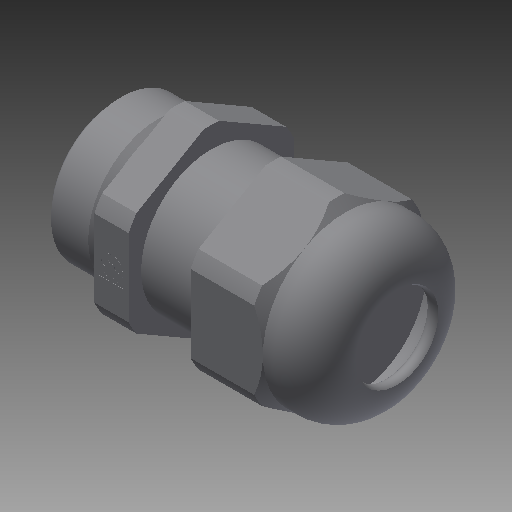
# Autodesk Inventor part: SKINTOP ST PG 13,5      Art. Nr. 53015030(F=5) Kunststoff
Saved by Autodesk Inventor 2019.3 (Build 233278000, 278)
## iProperties
Category: PARTsolutions
Company: LAPP
Created: 2018-12-13
Part Number: SKINTOP ST PG 13,5      Art. Nr. 53015030(F=5) Kunststoff
Material: Generic
Catalog Web Link: www.cadenas.de
Description: SKINTOP® ST-Cable gland plastic
Vendor: LAPP
Document SubType Name: Modeling
Designer: psadmin
Manufacturer: LAPP
Mass: 14.2643 g
Surface Area: 52.1864 cm^2
Volume: 14.2643 cm^3
Density: 1 g/cm^3
Appearance: PSOLRGB-175-175-175
PSOL_IDENT_0: {$CADENAS_DATA\23d-libs\lapp_kabel\skintop_kabelverschraubungen\skintop_kabelverschraubungen_polyami
PSOL_IDENT_1: d_pg\skintop_kabelverschraubungen_polyamid_pg\st_pg.prj},235 {VTYP=3D},{NB=SKINTOP ST PG 13,5      A
PSOL_IDENT_2: rt. Nr. 53015030(F=5)},{LINA=SKINTOP ST PG 13,5      Art. Nr. 53015030},{NN=SKINTOP® ST},{DATE=06.12
PSOL_IDENT_3: .2018 13:21:11},{GEOMDATE=18.12.2013 09:14:44},{VERSION=},{LINEID=100},{WBVAR=F},{WBNUMERIC=F}  {NB=
PSOL_IDENT_4: SKINTOP ST PG 13,5      Art. Nr. 53015030(F=5)},{LINA=SKINTOP ST PG 13,5      Art. Nr. 53015030},{KT=
PSOL_IDENT_5: DUMMY},{IDNR=},{ATN=53015030},{PG=PG 13,5},{ID=0.000},{RS=0.000},{FMIN=5.0},{FMAX=12.0},{F=5},{NDM=2
PSOL_IDENT_6: 0.4},{X=9},{SW=24},{A=26.5},{C=41.0},{D=9.0},{E=18.0},{H=10.5},{J=6.0},{K=5.0},{L=20.4},{XMAX=9},{RA
PSOL_IDENT_7: L7001=X},{RAL7035=},{RAL9005=},{MATERIAL=Kunststoff},{VPE=MIN}
NN: SKINTOP® ST
NT: Cable gland plastic
NB: SKINTOP® ST PG 13,5      Art. Nr. 53015030(F=5)
NBSYN: SKINTOP® ST $PG.      Art. Nr. $ATN.(F=$F.)
LINA: SKINTOP® ST PG 13,5      Art. Nr. 53015030
ATN: 53015030
PG: PG 13,5
FMIN: 5
FMAX: 12
F: 5
SW: 24
A: 26.5
C: 41
D: 9
RAL7001: X
MATERIAL: Plastic
VPE: 0
SUPPLIER: LAPP
ARTICLENO: SKINTOP ST PG 13,5      Art. Nr. 53015030(F=5)
BOMINFO: SKINTOP ST PG 13,5      Art. Nr. 53015030
CREATOR: CADENAS GmbH
Title: SKINTOP ST PG 13,5      Art. Nr. 53015030
Author: Cadenas PARTsolutions
Comments: Cable gland plastic
Autodesk Inventor part; units mm, degrees
ref_plane "YZ Plane" through (0, 0, 0) normal (1, 0, 0) x (0, 1, 0)
ref_plane "XZ Plane" through (0, 0, 0) normal (0, 1, 0) x (-1, 0, 0)
ref_plane "XY Plane" through (0, 0, 0) normal (0, 0, 1) x (1, 0, 0)
sketch "Sketch_1" plane through (0, 0, 0) normal (0, 0, 1) x (1, 0, 0)
  line L0 (41, 0) -> (0, 0)
  line L1 (0, 8.92) -> (0, 3.27)
  arc A0 (0, 3.27) -> (0.77, 2.5) centre (0.77, 3.27) ccw
  line L2 (0.77, 2.5) -> (35, 2.5)
  line L3 (35, 2.5) -> (35, 10.2)
  arc A1 (39.1884, 6.3116) -> (35, 10.2) centre (35, 6) ccw
  arc A2 (39.1884, 6.3116) -> (41, 6) centre (40.225, 6.9162) ccw
  arc A3 (41, 6) -> (35, 12) centre (35, 6) ccw
  line L4 (35, 12) -> (33.5, 12)
  line L5 (33.5, 12) -> (29.5, 16)
  line L6 (29.5, 16) -> (23, 16)
  line L7 (23, 16) -> (23, 10.2)
  line L8 (23, 10.2) -> (14, 10.2)
  line L9 (14, 10.2) -> (14, 16)
  line L10 (14, 16) -> (9, 16)
  line L11 (9, 16) -> (9, 9.69)
  line L12 (9, 9.69) -> (7.2, 9.69)
  line L13 (7.2, 9.69) -> (6.3167, 10.2)
  line L14 (6.3167, 10.2) -> (0.9, 10.2)
  line L15 (0.9, 10.2) -> (0.9, 9.69)
  line L16 (0.9, 9.69) -> (0.77, 9.69)
  arc A4 (0.77, 9.69) -> (0, 8.92) centre (0.77, 8.92) ccw
  constraints: 34 end point, 10 point on circle, 5 centre point
revolve "Revolution1" add sketch "Sketch_1" angle 360 about axis through (41, 0, 0) along (-1, 0, 0)
sketch "Sketch_2" plane through (9, 0, 0) normal (1, 0, 0) x (0, 0, -1)
  line L0 (-24, 24) -> (-24, -24)
  line L1 (-24, -24) -> (24, -24)
  line L2 (24, -24) -> (24, 24)
  line L3 (24, 24) -> (-24, 24)
  arc A0 (-12, -5.6181) -> (-10.8654, -7.5833) centre (0, 0) ccw
  line L4 (-10.8654, -7.5833) -> (-1.1346, -13.2013)
  arc A1 (-1.1346, -13.2013) -> (1.1346, -13.2013) centre (0, 0) ccw
  line L5 (1.1346, -13.2013) -> (10.8654, -7.5833)
  arc A2 (10.8654, -7.5833) -> (12, -5.6181) centre (0, 0) ccw
  line L6 (12, -5.6181) -> (12, 5.6181)
  arc A3 (12, 5.6181) -> (10.8654, 7.5833) centre (0, 0) ccw
  line L7 (10.8654, 7.5833) -> (1.1346, 13.2013)
  arc A4 (1.1346, 13.2013) -> (-1.1346, 13.2013) centre (0, 0) ccw
  line L8 (-1.1346, 13.2013) -> (-10.8654, 7.5833)
  arc A5 (-10.8654, 7.5833) -> (-12, 5.6181) centre (0, 0) ccw
  line L9 (-12, 5.6181) -> (-12, -5.6181)
  constraints: 20 end point, 12 point on circle, 6 centre point
extrude "Extrusion1" cut sketch "Sketch_2" along normal blind 41
sketch "Skizze_1" plane through (0, 0, 12) normal (0, 0, 1) x (1, 0, 0)
  line L0 (9.6667, 1.8333) -> (9.6667, -1.8333)
  line L1 (9.6667, -1.8333) -> (13.3333, -1.8333)
  line L2 (13.3333, -1.8333) -> (13.3333, 1.8333)
  line L3 (13.3333, 1.8333) -> (9.6667, 1.8333)
  arc A0 (9.8713, 0.3539) -> (10.3904, -1.2436) centre (11.5, 0) ccw
  line L4 (10.3904, -1.2436) -> (10.4659, -1.1398)
  arc A1 (10.7355, -1.3357) -> (10.4659, -1.1398) centre (10.9122, -0.809) ccw
  line L5 (10.7355, -1.3357) -> (10.6601, -1.4396)
  arc A2 (10.6601, -1.4396) -> (12.3399, -1.4396) centre (11.5, 0) ccw
  line L6 (12.3399, -1.4396) -> (12.2645, -1.3357)
  arc A3 (12.5341, -1.1398) -> (12.2645, -1.3357) centre (12.0878, -0.809) ccw
  line L7 (12.5341, -1.1398) -> (12.6096, -1.2436)
  arc A4 (12.6096, -1.2436) -> (13.1287, 0.3539) centre (11.5, 0) ccw
  line L8 (13.1287, 0.3539) -> (13.0066, 0.3143)
  arc A5 (12.9036, 0.6313) -> (13.0066, 0.3143) centre (12.4511, 0.309) ccw
  line L9 (12.9036, 0.6313) -> (13.0256, 0.671)
  arc A6 (13.0256, 0.671) -> (11.6667, 1.6583) centre (11.5, 0) ccw
  line L10 (11.6667, 1.6583) -> (11.6667, 1.53)
  arc A7 (11.3333, 1.53) -> (11.6667, 1.53) centre (11.5, 1) ccw
  line L11 (11.3333, 1.53) -> (11.3333, 1.6583)
  arc A8 (11.3333, 1.6583) -> (9.9744, 0.671) centre (11.5, 0) ccw
  line L12 (9.9744, 0.671) -> (10.0964, 0.6313)
  arc A9 (9.9934, 0.3143) -> (10.0964, 0.6313) centre (10.5489, 0.309) ccw
  line L13 (9.9934, 0.3143) -> (9.8713, 0.3539)
  constraints: 28 end point, 20 point on circle, 10 centre point
extrude "Extrusion2" cut sketch "Skizze_1" against normal blind 0.048
body "Solid1"
